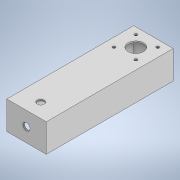
# Autodesk Inventor part: Soporte_base
Saved by Autodesk Inventor 2020 (Build 240168000, 168)
## iProperties
Created: 2023-03-22
Part Number: Soporte_base
Material: Generic
Document SubType Name: Modeling
Designer: semon
Density: 1 g/cm^3
Appearance: Default
Author: semon
Autodesk Inventor part; units mm, degrees
ref_plane "YZ Plane" through (0, 0, 0) normal (1, 0, 0) x (0, 1, 0)
ref_plane "XZ Plane" through (0, 0, 0) normal (0, 1, 0) x (-1, 0, 0)
ref_plane "XY Plane" through (0, 0, 0) normal (0, 0, 1) x (1, 0, 0)
sketch "Sketch1" plane through (0, 0, 0) normal (0, 0, 1) x (1, 0, 0)
  line L0 (-28, 0) -> (28, 0)
  line L1 (28, 0) -> (28, 40)
  line L2 (28, 40) -> (-28, 40)
  line L3 (-28, 40) -> (-28, 0)
  point P0 (0, 0)
  point P1 (0, 0)
  dimension "d1" = 56
  dimension "d2" = 40
  constraints: 8 end point, 2 parallel, 1 coincident, 1 horizontal, 1 midpoint, 1 perpendicular
  measures "d1" distance of L1.end L2.end
  measures "d2" distance of L0.end L1.end
extrude "Extrusion1" add sketch "Sketch1" along normal mid plane 180
shell "Shell1" thickness 2 removed faces 1 at (-9.3333, 0, 30)
sketch "Sketch2" plane through (0, 0, 90) normal (0, 0, 1) x (1, 0, 0)
  circle A0 centre (0, 20) radius 5
  line L0 (-28, 0) -> (28, 0) construction
  line L1 (28, 0) -> (28, 40) construction
  point P0 (0, 0)
  point P1 (0, 0)
  point P2 (28, 20)
  dimension "d6" = 10
  constraints: 2 midpoint, 1 centre point, 1 horizontal alignment, 1 vertical alignment
  measures "d6" diameter of A0
extrude "Extrusion2" cut sketch "Sketch2" against normal up to surface (2 mm away)
sketch "Sketch3" plane through (-28, 40, 90) normal (0, 1, 0) x (1, 0, 0)
  line L0 (56, 180) -> (56, 0) construction
  line L1 (56, 40) -> (0, 40) construction
  circle A0 centre (28, 155) radius 11
  circle A1 centre (12.5, 139.5) radius 2
  circle A2 centre (43.5, 170.5) radius 2
  circle A3 centre (12.5, 170.5) radius 2
  circle A4 centre (43.5, 139.5) radius 2
  line L2 (43.5, 139.5) -> (12.5, 139.5) construction
  line L3 (12.5, 139.5) -> (12.5, 170.5) construction
  line L4 (12.5, 170.5) -> (43.5, 170.5) construction
  line L5 (43.5, 170.5) -> (43.5, 139.5) construction
  line L6 (43.5, 139.5) -> (12.5, 170.5) construction
  line L7 (0, 0) -> (56, 0) construction
  line L8 (56, 0) -> (0, 40) construction
  line L9 (0, 180) -> (0, 0) construction
  circle A5 centre (28, 20) radius 5
  point P0 (28, 90)
  dimension "d9" = 40
  dimension "d10" = 4
  dimension "d11" = 22
  dimension "d12" = 115
  dimension "d13" = 31
  dimension "d16" = 10
  constraints: 14 end point, 6 centre point, 5 coincident, 3 equal radius, 2 horizontal, 2 midpoint, 2 parallel, 2 perpendicular, 2 point on line, 1 vertical alignment
  measures "d9" distance from line of L0.end L1
  measures "d10" diameter of A1
  measures "d11" diameter of A0
  measures "d12" distance from line of L1 A0.centre
  measures "d13" distance of L2.end L3.end
  measures "d16" diameter of A5
extrude "Extrusion3" cut sketch "Sketch3" against normal up to surface (2 mm away)
sketch "Sketch4" plane through (-28, 0, 90) normal (0, -1, 0) x (1, 0, 0)
  line L0 (2, -178) -> (2, -2) projected
  line L1 (54, -95) -> (2, -95)
  line L2 (2, -95) -> (2, -85)
  line L3 (2, -85) -> (54, -85)
  line L4 (54, -85) -> (54, -95)
  line L5 (54, -95) -> (2, -85) construction
  line L6 (2, -95) -> (54, -85) construction
  point P0 (28, -90)
  dimension "d17" = 10
  constraints: 12 end point, 2 midpoint, 2 parallel, 1 horizontal, 1 perpendicular, 1 point on line
  measures "d17" distance of L3.end L1.start
extrude "Extrusion4" add sketch "Sketch4" against normal blind 2
body "Solid2"
